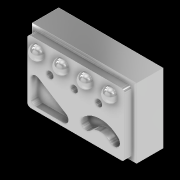
# Autodesk Inventor part: tarefa 3
Saved by Autodesk Inventor 2020 (Build 240168000, 168)
## iProperties
Created: 2021-01-13
Part Number: tarefa 3
Material: Generic
Document SubType Name: Modeling
Designer: Pedro Barriviera
Density: 1 g/cm^3
Appearance: Chrome - Polished
Author: Pedro Barriviera
Autodesk Inventor part; units mm, degrees
ref_plane "YZ Plane" through (0, 0, 0) normal (1, 0, 0) x (0, 1, 0)
ref_plane "XZ Plane" through (0, 0, 0) normal (0, 1, 0) x (-1, 0, 0)
ref_plane "XY Plane" through (0, 0, 0) normal (0, 0, 1) x (1, 0, 0)
sketch "Sketch1" plane through (0, 0, 0) normal (0, 0, 1) x (1, 0, 0)
  line L0 (0, 0) -> (150, 0)
  line L1 (150, 0) -> (150, 100)
  line L2 (150, 100) -> (0, 100)
  line L3 (0, 100) -> (0, 0)
  line L4 (5, 5) -> (145, 5)
  line L5 (145, 5) -> (145, 95)
  line L6 (145, 95) -> (5, 95)
  line L7 (5, 95) -> (5, 5)
  circle A0 centre (37.5, 60) radius 5
  line L8 (5, 60) -> (145, 60) construction
  circle A1 centre (72.5, 60) radius 5
  circle A2 centre (107.5, 60) radius 5
  arc A3 (10, 17) -> (17, 10) centre (17, 17) ccw
  arc A4 (57, 10) -> (60.71, 22.936) centre (57, 17) ccw
  arc A5 (20.71, 47.936) -> (10, 42) centre (17, 42) ccw
  line L9 (17, 10) -> (57, 10)
  line L10 (20.71, 47.936) -> (60.71, 22.936)
  line L11 (10, 17) -> (10, 42)
  circle A6 centre (130, 25) radius 8
  circle A7 centre (90, 25) radius 8
  line L12 (90, 25) -> (145, 25) construction
  arc A8 (124.2857, 19.4012) -> (95.7143, 19.4012) centre (110, 5.4041) ccw
  arc A9 (90.0041, 5) -> (90.0154, 4.6201) centre (110, 5.4041) ccw
  arc A10 (135.7143, 30.5988) -> (84.2857, 30.5988) centre (110, 5.4041) ccw
  dimension "d0" = 150
  dimension "d1" = 100
  dimension "d2" = 140
  dimension "d19" = 35
  dimension "d25" = 17
  dimension "d26" = 17
  dimension "d28" = 40
  dimension "d30" = 25
  dimension "d31" = 16
  dimension "d32" = 25
  dimension "d33" = 20
  dimension "d34" = 40
  dimension "d35" = 25
  dimension "d102" = 5
  dimension "d103" = 5
  dimension "d104" = 40
  dimension "d106" = 37.5
  dimension "d107" = 10
  dimension "d108" = 20
  dimension "d109" = 5
  dimension "d111" = 36
  dimension "d112" = 7
  dimension "d113" = 7
  dimension "d115" = 16
  dimension "d116" = 10
  dimension "d120" = 47.1699
  dimension "d121" = 40
  constraints: 26 end point, 16 point on circle, 11 centre point, 6 tangent, 5 point on line, 4 horizontal, 4 parallel, 3 perpendicular, 1 coincident, 1 vertical, 4 other
  measures "d0" distance of L2.end L1.end
  measures "d1" distance of L1.end L0.end
  measures "d2" distance of L6.end L5.end
  measures "d19" distance of A0.centre A1.centre
  measures "d25" distance from line of L3 A3.centre
  measures "d26" distance from line of L0 A3.centre
  measures "d28" distance of A4.centre A3.centre
  measures "d30" distance of A5.centre A3.centre
  measures "d31" diameter of A6
  measures "d32" distance from line of L0 A6.centre
  measures "d33" distance from line of L1 A6.centre
  measures "d34" distance of L12.start A6.centre
  measures "d35" distance from line of L0 L12.start
  measures "d102" distance between parallel lines of L3 L7
  measures "d103" distance between parallel lines of L2 L6
  measures "d104" distance from line of L2 A2.centre
  measures "d106" distance from line of L3 A0.centre
  measures "d107" diameter of A1
  measures "d108" radius of A8
  measures "d109" distance between parallel lines of L0 L4
  measures "d111" radius of A10
  measures "d112" radius of A5
  measures "d113" radius of A4
  measures "d115" diameter of A7
  measures "d116" distance between parallel lines of L3 L11
  measures "d120" distance of L10.start L10.end
  measures "d121" distance of L9.start L9.end
extrude "Extrusion1" add sketch "Sketch1" against normal blind 40 contours L3 L2 L1 L0 | L7 L6 L5 L4 | A0 | A1 | A2 | L11 A5 L10 A4 L9 A3 | A6 | A6 A8 A7 A10 | A7
extrude "Extrusion2" add sketch "Sketch1" along normal blind 10 contours L7 L6 L5 L4
extrude "Extrusion3" add sketch "Sketch1" along normal blind 10 contours A0 | A1 | A2
hole "Hole1" at (37.5, 60, 0) direction (0, 0, 1) diameter 10 end through all
hole "Hole2" at (72.5, 60, 0) direction (0, 0, 1) diameter 10 end through all
hole "Hole3" at (107.5, 60, 0) direction (0, 0, 1) diameter 10 end through all
hole "Hole4" at (37.5, 60, 0) direction (0, 0, -1) diameter 10 depth 13 tip angle 118
hole "Hole5" at (72.5, 60, 0) direction (0, 0, -1) diameter 10 depth 13 tip angle 118
hole "Hole6" at (107.5, 60, 0) direction (0, 0, -1) diameter 10 depth 13 tip angle 118
fillet "Fillet1" radius 5 1 edges at (145, 95, 5)
fillet "Fillet2" radius 5 3 edges at (5, 95, 5) (145, 5, 5) (5, 5, 5)
sketch "Sketch2" plane through (0, 0, 10) normal (0, 0, 1) x (1, 0, 0)
  arc A0 (30, 80) -> (10, 80) centre (20, 80) ccw
  line L0 (0, 100) -> (0, 0) projected
  line L1 (5, 10) -> (5, 90) construction
  line L2 (5, 80) -> (145, 80) construction
  line L3 (145, 90) -> (145, 10) construction
  line L4 (10, 80) -> (30, 80)
  arc A1 (65, 80) -> (45, 80) centre (55, 80) ccw
  line L5 (45, 80) -> (65, 80)
  arc A2 (100, 80) -> (80, 80) centre (90, 80) ccw
  line L6 (80, 80) -> (100, 80)
  arc A3 (135, 80) -> (115, 80) centre (125, 80) ccw
  line L7 (115, 80) -> (135, 80)
  dimension "d90" = 20
  dimension "d122" = 80
  dimension "d131" = 20
  dimension "d132" = 10
  dimension "d135" = 35
  constraints: 10 end point, 8 point on circle, 4 centre point, 4 point on line, 2 horizontal, 1 collinear, 15 other
  measures "d90" distance from line of L0 A0.centre
  measures "d122" vertical distance of L0.end A0.centre
  measures "d131" distance of L4.end L4.start
  measures "d132" radius of A0
  measures "d135" distance of A0.centre A1.centre
revolve "Revolution1" add sketch "Sketch2" angle 360 about axis through (5, 80, 10) along (1, 0, 0)
chamfer "Chamfer1" distance 2 angle 45 4 edges at (75, 100, 0) (150, 50, 0) (0, 50, 0) (75, 0, 0)
body "Solid1"
